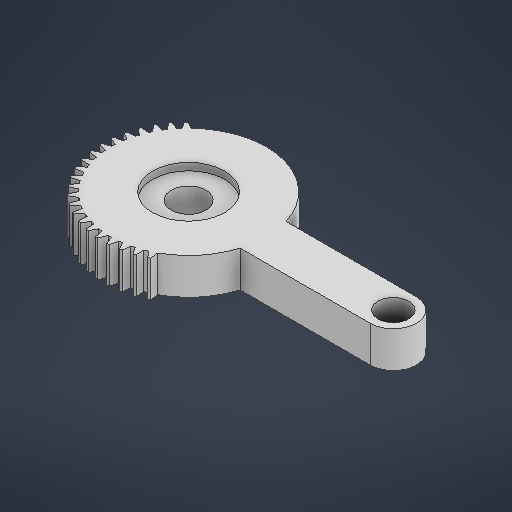
# Autodesk Inventor part: innerGear
Saved by Autodesk Inventor 2026.2 (Build 302298000, 298)
## iProperties
Created: 2026-04-07
Part Number: innerGear
Material: Generic
Document SubType Name: Modeling
Designer: Brian Wang
Density: 1 g/cm^3
Appearance: Default
Author: Brian Wang
Autodesk Inventor part; units mm, degrees
ref_plane "YZ Plane" through (0, 0, 0) normal (1, 0, 0) x (0, 1, 0)
ref_plane "XZ Plane" through (0, 0, 0) normal (0, 1, 0) x (-1, 0, 0)
ref_plane "XY Plane" through (0, 0, 0) normal (0, 0, 1) x (1, 0, 0)
sketch "Sketch1" plane through (0, 0, 0) normal (0, 1, 0) x (-1, 0, 0)
  circle A0 centre (0, 0) radius 11
  line L0 (0, 0) -> (21.5969, 0.9429) construction
  line L1 (0, 0) -> (22.384, -0.9773) construction
  line L2 (0, 0) -> (25.2479, 0) construction
  line L3 (10.9895, 0.4798) -> (12.0415, 0.1582)
  line L4 (10.9895, 0.4798) -> (12.0895, 0.4798) construction
  line L5 (10.9895, -0.4798) -> (12.0415, -0.1582)
  line L6 (12.0415, -0.1582) -> (12.0415, 0.1582)
  line L7 (10.9561, 0.9815) -> (11.9561, 1.4397)
  line L8 (11.9561, 1.4397) -> (11.9142, 1.7533)
  line L9 (10.8289, 1.9326) -> (11.9142, 1.7533)
  line L10 (10.7293, 2.4254) -> (11.6597, 3.0122)
  line L11 (11.6597, 3.0122) -> (11.5765, 3.3175)
  line L12 (10.4771, 3.3513) -> (11.5765, 3.3175)
  line L13 (10.313, 3.8266) -> (11.1574, 4.5315)
  line L14 (11.1574, 4.5315) -> (11.0345, 4.8231)
  line L15 (9.9402, 4.7109) -> (11.0345, 4.8231)
  line L16 (9.7146, 5.1602) -> (10.4581, 5.9708)
  line L17 (10.4581, 5.9708) -> (10.2976, 6.2435)
  line L18 (9.2279, 5.9872) -> (10.2976, 6.2435)
  line L19 (8.9446, 6.4026) -> (9.5741, 7.3047)
  line L20 (9.5741, 7.3047) -> (9.3789, 7.5537)
  line L21 (8.3526, 7.1578) -> (9.3789, 7.5537)
  line L22 (8.0168, 7.532) -> (8.521, 8.5096)
  line L23 (8.521, 8.5096) -> (8.2945, 8.7306)
  line L24 (7.3298, 8.2021) -> (8.2945, 8.7306)
  line L25 (6.9474, 8.5284) -> (7.3176, 9.5643)
  line L26 (7.3176, 9.5643) -> (7.0638, 9.7532)
  line L27 (6.1776, 9.1015) -> (7.0638, 9.7532)
  line L28 (5.7553, 9.3743) -> (5.9849, 10.45)
  line L29 (5.9849, 10.45) -> (5.7083, 10.6037)
  line L30 (4.9164, 9.8402) -> (5.7083, 10.6037)
  line L31 (4.4616, 10.0546) -> (4.5465, 11.1513)
  line L32 (4.5465, 11.1513) -> (4.252, 11.2669)
  line L33 (3.5683, 10.4052) -> (4.252, 11.2669)
  line L34 (3.0891, 10.5573) -> (3.0279, 11.6556)
  line L35 (3.0279, 11.6556) -> (2.7206, 11.7312)
  line L36 (2.1572, 10.7864) -> (2.7206, 11.7312)
  line L37 (1.6621, 10.8737) -> (1.4558, 11.9542)
  line L38 (1.4558, 11.9542) -> (1.1412, 11.9883)
  line L39 (0.708, 10.9772) -> (1.1412, 11.9883)
  line L40 (0.2057, 10.9981) -> (-0.142, 12.0417)
  line L41 (-0.142, 12.0417) -> (-0.4584, 12.0338)
  line L42 (-0.7536, 10.9742) -> (-0.4584, 12.0338)
  line L43 (-1.2543, 10.9283) -> (-1.7373, 11.9165)
  line L44 (-1.7373, 11.9165) -> (-2.0498, 11.8668)
  line L45 (-2.202, 10.7773) -> (-2.0498, 11.8668)
  line L46 (-2.6922, 10.6655) -> (-3.302, 11.581)
  line L47 (-3.302, 11.581) -> (-3.6051, 11.4902)
  line L48 (-3.6115, 10.3902) -> (-3.6051, 11.4902)
  line L49 (-4.0825, 10.2144) -> (-4.8083, 11.0409)
  line L50 (-4.8083, 11.0409) -> (-5.0967, 10.9108)
  line L51 (-4.9572, 9.8197) -> (-5.0967, 10.9108)
  line L52 (-5.4007, 9.5829) -> (-6.2297, 10.3059)
  line L53 (-6.2297, 10.3059) -> (-6.4983, 10.1387)
  line L54 (-6.2154, 9.0757) -> (-6.4983, 10.1387)
  line L55 (-6.6236, 8.7822) -> (-7.5411, 9.389)
  line L56 (-7.5411, 9.389) -> (-7.7852, 9.1876)
  line L57 (-7.3638, 8.1715) -> (-7.7852, 9.1876)
  line L58 (-7.7295, 7.8265) -> (-8.7194, 8.3062)
  line L59 (-8.7194, 8.3062) -> (-8.9346, 8.0743)
  line L60 (-8.3823, 7.1231) -> (-8.9346, 8.0743)
  line L61 (-8.699, 6.7326) -> (-9.7437, 7.0768)
  line L62 (-9.7437, 7.0768) -> (-9.9263, 6.8184)
  line L63 (-9.2527, 5.9488) -> (-9.9263, 6.8184)
  line L64 (-9.5148, 5.5198) -> (-10.596, 5.7225)
  line L65 (-10.596, 5.7225) -> (-10.7427, 5.4421)
  line L66 (-9.9597, 4.6695) -> (-10.7427, 5.4421)
  line L67 (-10.1627, 4.2095) -> (-11.2612, 4.2671)
  line L68 (-11.2612, 4.2671) -> (-11.3694, 3.9698)
  line L69 (-10.4909, 3.3078) -> (-11.3694, 3.9698)
  line L70 (-4.1308, 41.4833) -> (-4.8817, 42.2871)
  line L71 (-4.1308, 41.4833) -> (-4.6138, 42.4715) construction
  line L72 (-4.9929, 41.0618) -> (-5.1659, 42.1481)
  line L73 (-5.1659, 42.1481) -> (-4.8817, 42.2871)
  line L74 (-3.6939, 41.6623) -> (-3.7214, 42.762)
  line L75 (-3.7214, 42.762) -> (-3.4212, 42.862)
  line L76 (-2.7835, 41.9657) -> (-3.4212, 42.862)
  line L77 (-2.327, 42.0853) -> (-2.2084, 43.1789)
  line L78 (-2.2084, 43.1789) -> (-1.8976, 43.2383)
  line L79 (-1.3844, 42.2653) -> (-1.8976, 43.2383)
  line L80 (-0.9161, 42.3233) -> (-0.6536, 43.3915)
  line L81 (-0.6536, 43.3915) -> (-0.3377, 43.4091)
  line L82 (0.042, 42.3767) -> (-0.3377, 43.4091)
  line L83 (0.5138, 42.3721) -> (0.9156, 43.3961)
  line L84 (0.9156, 43.3961) -> (1.2311, 43.3717)
  line L85 (1.4705, 42.2981) -> (1.2311, 43.3717)
  line L86 (1.9373, 42.2309) -> (2.4714, 43.1926)
  line L87 (2.4714, 43.1926) -> (2.7808, 43.1266)
  line L88 (2.8758, 42.0307) -> (2.7808, 43.1266)
  line L89 (3.3295, 41.9023) -> (3.9864, 42.7847)
  line L90 (3.9864, 42.7847) -> (4.2843, 42.6782)
  line L91 (4.2332, 41.5794) -> (4.2843, 42.6782)
  line L92 (4.6657, 41.392) -> (5.4338, 42.1795)
  line L93 (5.4338, 42.1795) -> (5.715, 42.0345)
  line L94 (5.5186, 40.9521) -> (5.715, 42.0345)
  line L95 (5.9224, 40.7092) -> (6.788, 41.3879)
  line L96 (6.788, 41.3879) -> (7.0475, 41.2068)
  line L97 (6.7094, 40.1601) -> (7.0475, 41.2068)
  line L98 (7.0773, 39.8658) -> (8.0253, 40.4237)
  line L99 (8.0253, 40.4237) -> (8.2585, 40.2099)
  line L100 (7.7846, 39.2172) -> (8.2585, 40.2099)
  line L101 (8.1101, 38.8768) -> (9.1237, 39.3042)
  line L102 (9.1237, 39.3042) -> (9.3265, 39.0613)
  line L103 (8.7252, 38.1402) -> (9.3265, 39.0613)
  line L104 (9.0026, 37.7598) -> (10.064, 38.0489)
  line L105 (10.064, 38.0489) -> (10.2327, 37.7813)
  line L106 (9.5146, 36.9481) -> (10.2327, 37.7813)
  line L107 (9.7391, 36.5343) -> (10.8294, 36.6802)
  line L108 (10.8294, 36.6802) -> (10.9612, 36.3926)
  line L109 (10.1389, 35.662) -> (10.9612, 36.3926)
  line L110 (10.3066, 35.2222) -> (11.4066, 35.2223)
  line L111 (11.4066, 35.2223) -> (11.4991, 34.9197)
  line L112 (10.5872, 34.3045) -> (11.4991, 34.9197)
  line L113 (10.695, 33.8465) -> (11.7853, 33.7007)
  line L114 (11.7853, 33.7007) -> (11.8369, 33.3886)
  line L115 (10.8514, 32.8998) -> (11.8369, 33.3886)
  line L116 (10.8976, 32.4317) -> (11.9589, 32.1426)
  line L117 (11.9589, 32.1426) -> (11.9687, 31.8263)
  line L118 (10.9271, 31.4725) -> (11.9687, 31.8263)
  line L119 (10.9108, 31.0025) -> (11.9245, 30.5753)
  line L120 (11.9245, 30.5753) -> (11.8922, 30.2605)
  line L121 (10.8129, 30.0479) -> (11.8922, 30.2605)
  line L122 (10.7345, 29.5844) -> (11.6825, 29.0265)
  line L123 (11.6825, 29.0265) -> (11.6088, 28.7188)
  line L124 (10.5109, 28.6511) -> (11.6088, 28.7188)
  line L125 (10.3717, 28.2022) -> (11.2374, 27.5236)
  line L126 (11.2374, 27.5236) -> (11.1235, 27.2284)
  line L127 (10.0263, 27.3069) -> (11.1235, 27.2284)
  line L128 (9.8289, 26.8805) -> (10.597, 26.0931)
  line L129 (10.597, 26.0931) -> (10.445, 25.8156)
  line L130 (9.3679, 26.0389) -> (10.445, 25.8156)
  line L131 (9.1158, 25.6425) -> (9.7727, 24.7602)
  line L132 (9.7727, 24.7602) -> (9.5852, 24.5053)
  line L133 (8.5472, 24.8695) -> (9.5852, 24.5053)
  line L134 (8.2449, 24.5102) -> (8.779, 23.5485)
  line L135 (8.779, 23.5485) -> (8.5594, 23.3207)
  line L136 (7.5789, 23.8193) -> (8.5594, 23.3207)
  circle A1 centre (-28.0987, 31.6136) radius 2.125
  arc A2 (-28.0987, 34.7928) -> (-28.0987, 28.4345) centre (-28.0987, 31.6136) ccw
  line L137 (-28.0987, 34.7928) -> (-10.1175, 34.7928)
  line L138 (-28.0987, 28.4345) -> (-10.0978, 28.4345)
  line L139 (18.6565, 53.6502) -> (-47.4327, 53.6502)
  line L140 (18.6565, 53.6502) -> (84.7457, 53.6502) construction
  circle A3 centre (0.1722, 31.6106) radius 2.4
  arc A4 (-4.9929, 41.0618) -> (-10.1175, 34.7928) centre (0.1722, 31.6106) ccw
  arc A5 (-3.6939, 41.6623) -> (-4.1308, 41.4833) centre (0.1722, 31.6106) ccw
  arc A6 (-2.327, 42.0853) -> (-2.7835, 41.9657) centre (0.1722, 31.6106) ccw
  arc A7 (-0.9161, 42.3233) -> (-1.3844, 42.2653) centre (0.1722, 31.6106) ccw
  arc A8 (0.5138, 42.3721) -> (0.042, 42.3767) centre (0.1722, 31.6106) ccw
  arc A9 (1.9373, 42.2309) -> (1.4705, 42.2981) centre (0.1722, 31.6106) ccw
  arc A10 (3.3295, 41.9023) -> (2.8758, 42.0307) centre (0.1722, 31.6106) ccw
  arc A11 (4.6657, 41.392) -> (4.2332, 41.5794) centre (0.1722, 31.6106) ccw
  arc A12 (5.9224, 40.7092) -> (5.5186, 40.9521) centre (0.1722, 31.6106) ccw
  arc A13 (7.0773, 39.8658) -> (6.7094, 40.1601) centre (0.1722, 31.6106) ccw
  arc A14 (8.1101, 38.8768) -> (7.7846, 39.2172) centre (0.1722, 31.6106) ccw
  arc A15 (9.0026, 37.7598) -> (8.7252, 38.1402) centre (0.1722, 31.6106) ccw
  arc A16 (9.7391, 36.5343) -> (9.5146, 36.9481) centre (0.1722, 31.6106) ccw
  arc A17 (10.3066, 35.2222) -> (10.1389, 35.662) centre (0.1722, 31.6106) ccw
  arc A18 (10.695, 33.8465) -> (10.5872, 34.3045) centre (0.1722, 31.6106) ccw
  arc A19 (10.8976, 32.4317) -> (10.8514, 32.8998) centre (0.1722, 31.6106) ccw
  arc A20 (10.9108, 31.0025) -> (10.9271, 31.4725) centre (0.1722, 31.6106) ccw
  arc A21 (10.7345, 29.5844) -> (10.8129, 30.0479) centre (0.1722, 31.6106) ccw
  arc A22 (10.3717, 28.2022) -> (10.5109, 28.6511) centre (0.1722, 31.6106) ccw
  arc A23 (9.8289, 26.8805) -> (10.0263, 27.3069) centre (0.1722, 31.6106) ccw
  arc A24 (9.1158, 25.6425) -> (9.3679, 26.0389) centre (0.1722, 31.6106) ccw
  arc A25 (-10.0978, 28.4345) -> (7.5789, 23.8193) centre (0.1722, 31.6106) ccw
  arc A26 (8.2449, 24.5102) -> (8.5472, 24.8695) centre (0.1722, 31.6106) ccw
  dimension "d0" = 22
  dimension "d1" = 2.5
  dimension "d2" = 2.5
  dimension "d3" = 1.1
  dimension "d4" = 17
  dimension "d5" = 0.3164
  dimension "d8" = 160
  dimension "d12" = 4.25
  dimension "d16" = 4.8
  dimension "d21" = 10.75
  constraints: 282 end point, 48 point on circle, 45 point on line, 26 centre point, 4 coincident, 4 horizontal, 2 equal length, 2 symmetric about line, 2 tangent, 1 parallel, 1 vertical, 172 other
  measures "d1" angle of L2 L0
  measures "d2" angle of L1 L2
  measures "d3" distance of L3.start L3.end
  measures "d4" angle of L3 L4
  measures "d5" distance of L5.end L6.end
  measures "d12" diameter of A1
  measures "d16" diameter of A3
  measures "d21" radius of A25
extrude "Extrusion1" add sketch "Sketch1" along normal blind 5 contours A5 L74 L75 L76 A6 L77 L78 L79 A7 L80 L81 L82 A8 L83 L84 L85 A9 L86 L87 L88 A10 L89 L90 L91 A11 L92 L93 L94 A12 L95 L96 L97 A13 L98 L99 L100 A14 L101 L102 L103 A15 L104 L105 L106 A16 L107 L108 L109 A17 L110 L111 L112 A18 L113 L114 L115 A19 L116 L117 L118 A20 L119 L120 L121 A21 L122 L123 L124 A22 L125 L126 L127 A23 L128 L129 L130 A24 L131 L132 L133 A26 L134 L135 L136 A25 L138 A2 L137 A4 L72 L73 L70
sketch "Sketch2" plane through (0, 5, 0) normal (0, 1, 0) x (1, 0, 0)
  circle A0 centre (-0.1722, -31.6106) radius 2.4 projected
  circle A1 centre (-0.1722, -31.6106) radius 4.9724
  point P0 (0, 0)
  constraints: 1 centre point, 1 coincident
extrude "Extrusion2" cut sketch "Sketch2" against normal blind 1
body "Solid1"
